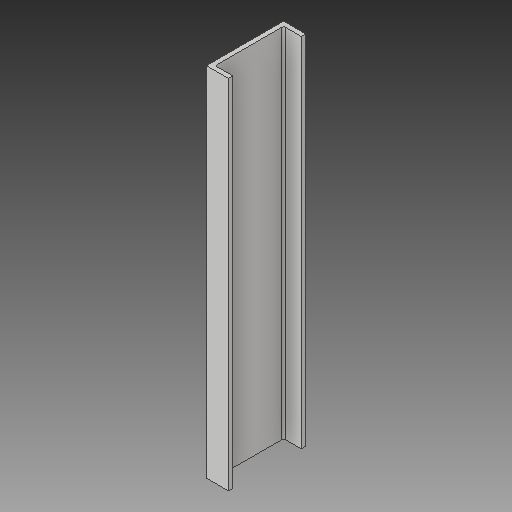
# Autodesk Inventor part: Base1
Saved by Autodesk Inventor 2019 (Build 230136000, 136)
## iProperties
Created: 2019-07-01
Part Number: Base1
Material: Generic
Document SubType Name: Sheet Metal
Designer: Satwik Pandey
Density: 1 g/cm^3
Sheet Metal Rule: Default_mm
Appearance: Default
Author: Satwik Pandey
Autodesk Inventor part; units mm, degrees
ref_plane "YZ Plane" through (0, 0, 0) normal (1, 0, 0) x (0, 1, 0)
ref_plane "XZ Plane" through (0, 0, 0) normal (0, 1, 0) x (-1, 0, 0)
ref_plane "XY Plane" through (0, 0, 0) normal (0, 0, 1) x (1, 0, 0)
sketch "Sketch1" plane through (0, 0, 0) normal (1, 0, 0) x (0, 1, 0)
  line L0 (0, 0) -> (810, 0)
  line L1 (810, 0) -> (810, -175)
  line L2 (810, -175) -> (0, -175)
  line L3 (0, -175) -> (0, 0)
  constraints: 8 end point, 2 parallel, 1 horizontal, 1 perpendicular
extrude "Extrusion1" add sketch "Sketch1" along normal blind 10
sketch "Sketch2" plane through (10, 0, 0) normal (1, 0, 0) x (0, 0, -1)
  line L0 (0, 810) -> (0, 0) projected
  line L1 (175, 0) -> (175, 810) projected
  line L2 (0, 0) -> (175, 0)
  line L3 (175, 0) -> (175, 10)
  line L4 (175, 10) -> (0, 10)
  line L5 (0, 10) -> (0, 0)
  line L6 (175, 810) -> (0, 810) projected
  line L7 (0, 10) -> (10, 10)
  line L8 (10, 10) -> (10, 810)
  line L9 (10, 810) -> (0, 810)
  line L10 (0, 810) -> (0, 10)
  line L11 (10, 810) -> (175, 810)
  line L12 (175, 810) -> (175, 800)
  line L13 (175, 800) -> (10, 800)
  line L14 (10, 800) -> (10, 810)
  line L15 (175, 800) -> (165, 800)
  line L16 (165, 800) -> (165, 10)
  line L17 (165, 10) -> (175, 10)
  line L18 (175, 10) -> (175, 800)
  dimension "d4" = 10
  dimension "d5" = 10
  dimension "d6" = 10
  dimension "d7" = 10
  constraints: 32 end point, 8 parallel, 4 horizontal, 4 perpendicular, 4 point on line
  measures "d4" distance of L3.end L2.end
  measures "d5" distance of L9.end L8.end
  measures "d6" distance of L11.end L12.end
  measures "d7" distance of L17.end L16.end
extrude "Extrusion2" add sketch "Sketch2" along normal blind 40
sketch "Sketch3" plane through (50, 0, 0) normal (1, 0, 0) x (0, 0, -1)
  line L0 (175, 0) -> (0, 0) projected
  line L1 (0, 810) -> (175, 810) projected
  line L2 (10, 0) -> (165, 0)
  line L3 (165, 0) -> (165, 810)
  line L4 (165, 810) -> (10, 810)
  line L5 (10, 810) -> (10, 0)
  dimension "d10" = 155
  constraints: 8 end point, 2 parallel, 2 point on line, 1 horizontal, 1 perpendicular
  measures "d10" distance of L4.end L3.end
extrude "Extrusion3" cut sketch "Sketch3" against normal blind 40
fillet "Fillet1" radius 4 1 edges at (10, 405, -165)
fillet "Fillet2" radius 4 1 edges at (10, 405, -10)
equation "\"BendRadius\" = Thickness"
equation "\"BendReliefWidth\" = Thickness"
equation "\"BendReliefDepth\" = 0.5 * Thickness"
equation "\"CornerReliefSize\" = 4 * Thickness"
equation "\"MinimumRemnant\" = 2 * Thickness"
equation "\"TransitionRadius\" = BendRadius"
equation "\"JacobiRadiusSize\" = BendRadius"
equation "\"GapSize\" = Thickness"
equation "\"Thickness\" = 0.5"
body "Solid1"
